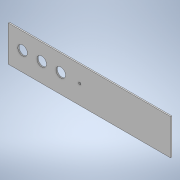
# Autodesk Inventor part: 220207 Front Bottom
Saved by Autodesk Inventor 2022 (Build 260153000, 153)
## iProperties
Created: 2022-02-07
Part Number: 220207 Front Bottom
Material: Generic
Document SubType Name: Modeling
Designer: josephinew
Density: 1 g/cm^3
Appearance: Default
Author: josephinew
Autodesk Inventor part; units mm, degrees
ref_plane "YZ Plane" through (0, 0, 0) normal (1, 0, 0) x (0, 1, 0)
ref_plane "XZ Plane" through (0, 0, 0) normal (0, 1, 0) x (-1, 0, 0)
ref_plane "XY Plane" through (0, 0, 0) normal (0, 0, 1) x (1, 0, 0)
sketch "Sketch1" plane through (0, 0, 0) normal (0, 0, 1) x (1, 0, 0)
  line L0 (0, 0) -> (431.8, 0)
  line L1 (431.8, 0) -> (431.8, 95.25)
  line L2 (431.8, 95.25) -> (0, 95.25)
  line L3 (0, 95.25) -> (0, 0)
  dimension "d0" = 431.8
  dimension "d1" = 95.25
  constraints: 8 end point, 2 parallel, 1 horizontal, 1 perpendicular
  measures "d0" distance of L2.end L1.end
  measures "d1" distance of L1.end L0.end
extrude "Extrusion1" add sketch "Sketch1" along normal blind 3.175
sketch "Sketch2" plane through (0, 0, 3.175) normal (0, 0, 1) x (1, 0, 0)
  line L0 (0, 0) -> (38.1, 0)
  line L1 (0, 50.8) -> (0, 0)
  circle A0 centre (38.1, 50.8) radius 12.7
  circle A1 centre (88.9, 50.8) radius 12.7
  circle A2 centre (139.7, 50.8) radius 12.7
  circle A3 centre (190.5, 50.8) radius 3.048
  dimension "d6" = 25.4
  dimension "d18" = 6.096
  constraints: 4 centre point, 4 end point, 1 horizontal
  measures "d6" diameter of A0
  measures "d18" diameter of A3
extrude "Extrusion2" cut sketch "Sketch2" against normal blind 25.4
body "Solid1"
